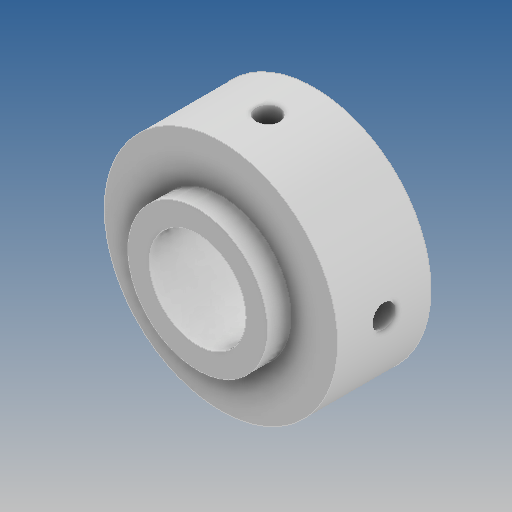
# Autodesk Inventor part: 0008-30-008
Saved by Autodesk Inventor 2020 (Build 240168000, 168)
## iProperties
Created: 2021-05-24
Part Number: 0008-30-008
Material: Generic
Document SubType Name: Modeling
Designer: Iulian Bors
Density: 1 g/cm^3
Appearance: Default
Author: Iulian Bors
Subject: 008
Autodesk Inventor part; units mm, degrees
ref_plane "YZ Plane" through (0, 0, 0) normal (1, 0, 0) x (0, 1, 0)
ref_plane "XZ Plane" through (0, 0, 0) normal (0, 1, 0) x (-1, 0, 0)
ref_plane "XY Plane" through (0, 0, 0) normal (0, 0, 1) x (1, 0, 0)
sketch "Sketch1" plane through (0, 0, 0) normal (0, 0, 1) x (1, 0, 0)
  circle A0 centre (0, 0) radius 4.15
  circle A1 centre (0, 0) radius 10
  dimension "d0" = 8.3
  dimension "d1" = 20
  constraints: 2 centre point, 2 coincident
  measures "d0" diameter of A0
  measures "d1" diameter of A1
extrude "Extrusion1" add sketch "Sketch1" along normal blind 10
sketch "Sketch2" plane through (0, 0, 0) normal (1, 0, 0) x (0, 1, 0)
  line L0 (10, 0) -> (10, 10) projected
  line L1 (10, 0) -> (-10, 0) projected
  point P0 (0, 0)
  point P1 (0, 4)
  dimension "d22" = 4
  constraints: 1 vertical alignment
  measures "d22" distance from line of L1 point (0, 4)
hole "Hole1" at (0, 0, 4) direction (-1, 0, 0) diameter 2 end through all both
sketch "Sketch3" plane through (0, 0, 0) normal (0, 1, 0) x (-1, 0, 0)
  line L0 (10, 0) -> (-10, 0) projected
  point P0 (0, 0)
  point P1 (0, 4)
  dimension "d11" = 4
  constraints: 1 vertical alignment
  measures "d11" distance from line of L0 point (0, 4)
hole "Hole2" at (0, 0, 4) direction (0, 1, 0) diameter 2 end through all both
sketch "Sketch4" plane through (0, 0, 10) normal (0, 0, 1) x (1, 0, 0)
  circle A0 centre (0, 0) radius 10 projected
  circle A1 centre (0, 0) radius 4.15 projected
  circle A2 centre (0, 0) radius 6
  dimension "d21" = 12
  constraints: 1 centre point, 1 coincident
  measures "d21" diameter of A2
extrude "Extrusion2" cut sketch "Sketch4" against normal blind 2 contours A0
body "Solid1"
